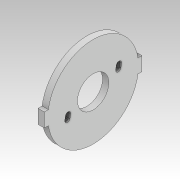
# Autodesk Inventor part: ValvePlate
Saved by Autodesk Inventor 2020 (Build 240168000, 168)
## iProperties
Created: 2021-10-11
Part Number: ValvePlate
Material: Generic
Document SubType Name: Modeling
Designer: DDeGo
Density: 1 g/cm^3
Appearance: Default
Author: DDeGo
Autodesk Inventor part; units mm, degrees
ref_plane "YZ Plane" through (0, 0, 0) normal (1, 0, 0) x (0, 1, 0)
ref_plane "XZ Plane" through (0, 0, 0) normal (0, 1, 0) x (-1, 0, 0)
ref_plane "XY Plane" through (0, 0, 0) normal (0, 0, 1) x (1, 0, 0)
sketch "Sketch1" plane through (0, 0, 0) normal (1, 0, 0) x (0, 1, 0)
  circle A0 centre (0, 0) radius 13
  line L0 (-2, -14) -> (2, -14)
  line L1 (2, -14) -> (2, 14)
  line L2 (2, 14) -> (-2, 14)
  line L3 (-2, 14) -> (-2, -14)
  line L4 (-2, -14) -> (2, 14) construction
  line L5 (2, -14) -> (-2, 14) construction
  circle A1 centre (0, 0) radius 4.5
  point P0 (2, -12.8452)
  point P1 (2, 12.8452)
  point P2 (-2, 12.8452)
  point P3 (-2, -12.8452)
  dimension "d0" = 4
  dimension "d1" = 26
  dimension "d2" = 28
  dimension "d5" = 9
  constraints: 12 end point, 2 centre point, 2 coincident, 2 midpoint, 2 parallel, 1 horizontal, 1 perpendicular
  measures "d0" distance of L1.end L2.end
  measures "d1" diameter of A0
  measures "d2" distance of L0.end L1.end
  measures "d5" diameter of A1
extrude "Extrusion1" add sketch "Sketch1" along normal blind 1.8 contours A0 L1 A1 | L1 A1 L3 A0 | A0 L3 L2 L1 | L1 L0 L3 A0 | A0 L3 A1 L1 | L3 A1 A0
sketch "Sketch2" plane through (1.8, 0, 0) normal (1, 0, 0) x (0, 0, -1)
  line L0 (7.4, 3.2) -> (7.2, 2.1) construction
  line L1 (6.6621, 3.3342) -> (6.4621, 2.2342)
  line L2 (7.9379, 1.9658) -> (8.1379, 3.0658)
  arc A0 (8.1379, 3.0658) -> (6.6621, 3.3342) centre (7.4, 3.2) ccw
  arc A1 (6.4621, 2.2342) -> (7.9379, 1.9658) centre (7.2, 2.1) ccw
  point P0 (0, 0)
  point P1 (7.3, 2.65)
  dimension "d6" = 0.75
  dimension "d9" = 7.2
  dimension "d10" = 2.1
  dimension "d11" = 7.4
  dimension "d12" = 3.2
  constraints: 8 end point, 4 point on circle, 4 tangent, 2 centre point, 1 midpoint, 1 parallel
  measures "d6" radius of A1
  measures "d9" horizontal distance of point (0, 0) L0.end
  measures "d10" vertical distance of point (0, 0) L0.end
  measures "d11" horizontal distance of point (0, 0) L0.start
  measures "d12" vertical distance of point (0, 0) L0.start
extrude "Extrusion2" cut sketch "Sketch2" against normal blind 1.3
sketch "Sketch3" plane through (0, 0, 0) normal (-1, 0, 0) x (0, 0, 1)
  arc A0 (-7.9379, 1.9658) -> (-6.4621, 2.2342) centre (-7.2, 2.1) ccw construction
  line L0 (-8.1379, 3.0658) -> (-7.9379, 1.9658) construction
  arc A1 (-6.6621, 3.3342) -> (-8.1379, 3.0658) centre (-7.4, 3.2) ccw construction
  line L1 (-6.4621, 2.2342) -> (-6.6621, 3.3342) construction
  circle A2 centre (0, 0) radius 9 construction
  line L2 (-7.4, 3.2) -> (-7.2, 2.1) construction
  circle A3 centre (-9.5, 5.5) radius 1
  dimension "d13" = 18
  dimension "d17" = 9.5
  dimension "d18" = 5.5
  dimension "d19" = 2
  constraints: 2 centre point, 2 end point, 1 coincident
  measures "d13" diameter of A2
  measures "d17" horizontal distance of point (0, 0) A3.centre
  measures "d18" vertical distance of point (0, 0) A3.centre
  measures "d19" diameter of A3
extrude "Extrusion3" cut sketch "Sketch3" against normal blind 1.3
sketch "Sketch4" plane through (1.3, 5.5, -9.5) normal (-1, 0, 0) x (0, 0, 1)
  circle A0 centre (0, 0) radius 1 projected
  arc A1 (1.5621, -3.5342) -> (3.0379, -3.2658) centre (2.3, -3.4) ccw projected
  line L0 (1.3621, -2.4342) -> (1.5621, -3.5342) projected
  arc A2 (2.8379, -2.1658) -> (1.3621, -2.4342) centre (2.1, -2.3) ccw projected
  line L1 (3.0379, -3.2658) -> (2.8379, -2.1658) projected
  line L2 (0.7902, 0.6128) -> (2.6927, -1.8404)
  arc A3 (2.8379, -2.1658) -> (1.3621, -2.4342) centre (2.1, -2.3) ccw projected
  circle A4 centre (0, 0) radius 1 projected
  line L3 (-0.7926, -0.6097) -> (1.7055, -3.8573)
  arc A5 (1.5621, -3.5342) -> (3.0379, -3.2658) centre (2.3, -3.4) ccw projected
  circle A6 centre (0, 0) radius 1 projected
  point P0 (9.5, -5.5)
  point P1 (2.6927, -1.8404)
  point P2 (-0.7926, -0.6097)
  constraints: 4 end point, 4 tangent, 3 point on circle, 2 other
extrude "Extrusion4" cut sketch "Sketch4" along normal up to surface (0.8 mm away) contours A0 L2 A2 L0 A1 L3
pattern_circular "Circular Pattern1" count 2 over 360 about axis through (0, 0, 0) along (1, 0, 0) of "Extrusion2", "Extrusion3", "Extrusion4"
body "Solid1"
